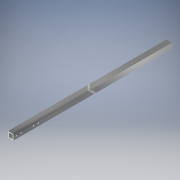
# Autodesk Inventor part: 15102898-16-P-0216
Saved by Autodesk Inventor 2017 (Build 210142000, 142)
## iProperties
Created: 2016-10-06
Part Number: 15102898-16-P-0216
Material: Aluminum 6061
Document SubType Name: Modeling
Designer: gus
Density: 2.7 g/cm^3
Appearance: Aluminum - Flat
Author: gus
Autodesk Inventor part; units mm, degrees
ref_plane "YZ Plane" through (0, 0, 0) normal (1, 0, 0) x (0, 1, 0)
ref_plane "XZ Plane" through (0, 0, 0) normal (0, 1, 0) x (-1, 0, 0)
ref_plane "XY Plane" through (0, 0, 0) normal (0, 0, 1) x (1, 0, 0)
sketch "Sketch1" plane through (0, 0, 0) normal (0, 0, 1) x (1, 0, 0)
  line L0 (0, 0) -> (-25.4, 0)
  line L1 (-25.4, 0) -> (-25.4, 25.4)
  line L2 (-25.4, 25.4) -> (0, 25.4)
  line L3 (0, 25.4) -> (0, 0)
  line L4 (-22.225, 22.225) -> (-22.225, 3.175)
  line L5 (-22.225, 3.175) -> (-3.175, 3.175)
  line L6 (-3.175, 3.175) -> (-3.175, 22.225)
  line L7 (-3.175, 22.225) -> (-22.225, 22.225)
  dimension "d0" = 25.4
  dimension "d1" = 25.4
  dimension "d2" = 3.175
  constraints: 16 end point, 4 parallel, 2 perpendicular, 1 horizontal, 3 other
  measures "d0" distance of L1.end L2.end
  measures "d1" distance of L0.end L1.end
  measures "d2" distance between parallel lines of L1 L4
extrude "Extrusion1" add sketch "Sketch1" along normal blind 736.6
sketch "Sketch2" plane through (-25.4, 25.4, 0) normal (0, 1, 0) x (1, 0, 0)
  circle A0 centre (12.7, -177.8) radius 3.175
  line L0 (0, 0) -> (0, -736.6) projected
  line L1 (0, 0) -> (25.4, 0) projected
  dimension "d5" = 6.35
  dimension "d6" = 12.7
  dimension "d7" = 177.8
  constraints: 1 centre point
  measures "d5" diameter of A0
  measures "d6" distance from line of L0 A0.centre
  measures "d7" distance from line of L1 A0.centre
extrude "Extrusion2" cut sketch "Sketch2" against normal blind 25.4
sketch "Sketch3" plane through (-25.4, 0, 0) normal (-1, 0, 0) x (0, 0, 1)
  circle A0 centre (723.9, 12.7) radius 3.175
  line L0 (0, 0) -> (736.6, 0) projected
  line L1 (736.6, 25.4) -> (736.6, 0) projected
  line L2 (736.6, 12.7) -> (584.2, 12.7) construction
  circle A1 centre (701.675, 12.7) radius 3.175
  circle A2 centre (644.525, 12.7) radius 3.175
  circle A3 centre (622.3, 12.7) radius 3.175
  dimension "d10" = 6.35
  dimension "d11" = 12.7
  dimension "d12" = 152.4
  dimension "d13" = 12.7
  dimension "d14" = 12.7
  dimension "d15" = 6.35
  dimension "d16" = 22.225
  dimension "d17" = 6.35
  dimension "d18" = 6.35
  dimension "d19" = 57.15
  dimension "d20" = 22.225
  constraints: 4 centre point, 3 point on line, 2 end point, 1 horizontal, 1 midpoint
  measures "d10" diameter of A0
  measures "d11" distance from line of L0 A0.centre
  measures "d12" distance of L2.start L2.end
  measures "d13" distance between parallel lines of L0 L2
  measures "d14" distance from line of L1 A0.centre
  measures "d15" diameter of A1
  measures "d16" distance of A0.centre A1.centre
  measures "d17" diameter of A2
  measures "d18" diameter of A3
  measures "d19" distance of A1.centre A2.centre
  measures "d20" distance of A3.centre A2.centre
extrude "Extrusion3" cut sketch "Sketch3" against normal blind 25.4
body "Solid1"
